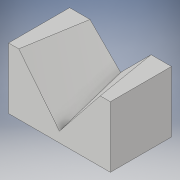
# Autodesk Inventor part: AW5.5bloft
Saved by Autodesk Inventor 2018 (Build 220112000, 112)
## iProperties
Created: 2019-01-22
Part Number: AW5.5bloft
Material: Generic
Document SubType Name: Modeling
Designer: russd
Density: 1 g/cm^3
Appearance: Default
Author: russd
Autodesk Inventor part; units mm, degrees
ref_plane "YZ Plane" through (0, 0, 0) normal (1, 0, 0) x (0, 1, 0)
ref_plane "XZ Plane" through (0, 0, 0) normal (0, 1, 0) x (-1, 0, 0)
ref_plane "XY Plane" through (0, 0, 0) normal (0, 0, 1) x (1, 0, 0)
sketch "Sketch1" plane through (0, 0, 0) normal (0, 0, 1) x (1, 0, 0)
  line L0 (-13.5055, 7.2192) -> (49.9945, 7.2192)
  line L1 (49.9945, 7.2192) -> (49.9945, -30.8808)
  line L2 (49.9945, -30.8808) -> (-13.5055, -30.8808)
  line L3 (-13.5055, -30.8808) -> (-13.5055, 7.2192)
  point P0 (0, 0)
  dimension "d0" = 63.5
  dimension "d1" = 38.1
  constraints: 8 end point, 2 parallel, 1 horizontal, 1 perpendicular
  measures "d0" distance of L1.end L2.end
  measures "d1" distance of L0.end L1.end
extrude "Extrusion1" add sketch "Sketch1" along normal blind 38.1
sketch "Sketch2" plane through (0, 0, 38.1) normal (0, 0, 1) x (1, 0, 0)
  line L0 (18.2445, -24.5308) -> (43.6445, 7.2192)
  line L1 (49.9945, 7.2192) -> (-13.5055, 7.2192) projected
  line L2 (18.2445, -24.5308) -> (-7.1555, 7.2192)
  line L3 (-13.5055, -30.8808) -> (49.9945, -30.8808) projected
  point P0 (0, 0)
  dimension "d4" = 6.35
  dimension "d5" = 6.35
  dimension "d6" = 6.35
  constraints: 4 end point, 2 point on line, 1 equal length
  measures "d4" distance from line of L0.start L3
  measures "d5" distance of L1.start L0.end
  measures "d6" distance of L2.end L1.end
sketch "Sketch4" plane through (0, 0, 0) normal (0, 0, -1) x (-1, 0, 0)
  line L0 (-18.2445, -11.8308) -> (-37.2945, 7.2192)
  line L1 (-49.9945, 7.2192) -> (13.5055, 7.2192) projected
  line L2 (-18.2445, -11.8308) -> (0.8055, 7.2192)
  line L3 (-49.9945, -30.8808) -> (13.5055, -30.8808) projected
  point P0 (0, 0)
  dimension "d8" = 19.05
  dimension "d9" = 12.7
  dimension "d10" = 12.7
  constraints: 4 end point, 2 point on line, 1 perpendicular
  measures "d8" distance from line of L3 L0.start
  measures "d9" distance of L1.end L2.end
  measures "d10" distance of L0.end L1.start
loft "Loft1" cut profiles "Sketch4", "Sketch2"
body "Solid1"
